Autodesk Fusion 360 part; units mm, degrees
(part 6 of 6)
equation "ChamberRear = CaseDepth - Cover - 2.8 mm" comment "Rear of closed sampling cartridge"
equation "ChamberLid = 2 mm" comment "Independent internal chamber lid"
equation "ChamberSideX = 45.6 mm" comment "Start of viewer-left vertical gas chamber column"
equation "ChamberLeft = 2.9 mm" comment "Upper chamber inner-case margin"
equation "ChamberRight = CaseWidth - 2.9 mm" comment "Upper and side chamber extent"
equation "ChamberBottom = 30 mm" comment "Lower gas column clears USB mounting region"
equation "ChamberTop = CaseHeight - 2.9 mm" comment "Top clearance to housing"
equation "ChamberBarY = 87 mm" comment "Lower edge of horizontal upper gas chamber"
equation "GasY = 105 mm" comment "Upper cross-flow port height"
equation "GasZ = 23 mm" comment "Side-fitting depth centre"
equation "GasBore = 2.5 mm" comment "5 mm ID nominal sample ports"
equation "UsbY = 16 mm" comment "Low on viewer-left side, below gas column"
equation "UsbZ = 27 mm" comment "USB connector centre depth"
equation "ButtonY = 45 mm" comment "Right-side power button, behind holder"
equation "ButtonZ = 44.5 mm" comment "Button clearance behind measured thin holder"
equation "d45 = CaseWidth"
equation "d46 = CaseHeight"
equation "d47 = CaseDepth - Cover"
equation "d49 = RearInset"
equation "d50 = RearInset"
equation "d51 = CaseWidth - 2 * RearInset"
equation "d52 = CaseHeight - 2 * RearInset"
equation "d54 = CornerRadius"
equation "d57 = Wall"
equation "d58 = Wall"
equation "d59 = CaseWidth - 2 * Wall"
equation "d60 = CaseHeight - 2 * Wall"
equation "d61 = CaseDepth"
equation "d64 = CornerRadius - Wall"
equation "d67 = DisplayX - DisplayFit"
equation "d68 = DisplayY - DisplayFit"
equation "d69 = DisplayWidth + 2 * DisplayFit"
equation "d70 = DisplayHeight + 2 * DisplayFit"
equation "d75 = -( -( GasZ ) )"
equation "d76 = GasY"
equation "d78 = CaseWidth + 2 mm"
equation "d82 = -( -( ButtonZ ) )"
equation "d83 = ButtonY"
equation "d85 = Wall + 2 mm"
equation "d87 = CaseWidth - Wall - 1 mm"
equation "d89 = -( -( ( UsbZ - 8 mm ) + ( 16 mm ) ) )"
equation "d90 = UsbY - 10 mm"
equation "d93 = Wall + 2 mm"
equation "d95 = CaseDepth - Cover + CoverGap"
equation "d97 = RearInset"
equation "d98 = RearInset"
equation "d99 = CaseWidth - 2 * RearInset"
equation "d100 = CaseHeight - 2 * RearInset"
equation "d101 = Cover - CoverGap"
equation "d104 = CornerRadius"
equation "d105 = DisplayFront"
equation "d107 = DisplayX"
equation "d108 = DisplayY"
equation "d109 = DisplayWidth"
equation "d110 = DisplayHeight"
equation "d111 = DisplayDepth"
equation "d115 = DisplayFront + 3 mm"
equation "d117 = CaseWidth / 2 - 32.7 mm"
equation "d118 = CaseHeight / 2 - 54 mm"
equation "d123 = DisplayFront - 0.1 mm"
equation "d125 = ( CaseWidth - GlassWidth ) / 2"
equation "d126 = ( CaseHeight - GlassHeight ) / 2"
equation "d127 = GlassWidth"
equation "d128 = GlassHeight"
equation "d131 = DisplayFront"
equation "d133 = ( CaseWidth - GlassWidth ) / 2"
equation "d134 = ( CaseHeight - GlassHeight ) / 2"
equation "d135 = GlassWidth"
equation "d136 = GlassHeight"
equation "d139 = DisplayFront - 0.1 mm"
equation "d141 = ( CaseWidth - ActiveWidth ) / 2"
equation "d142 = ( CaseHeight - ActiveHeight ) / 2"
equation "d143 = ActiveWidth"
equation "d144 = ActiveHeight"
equation "d147 = DisplayFront"
equation "d149 = ( CaseWidth - ActiveWidth ) / 2"
equation "d150 = ( CaseHeight - ActiveHeight ) / 2"
equation "d151 = ActiveWidth"
equation "d152 = ActiveHeight"
equation "d157 = CaseWidth / 2 - 32.53 mm"
equation "d158 = CaseHeight / 2 - 54 mm"
equation "d165 = CaseWidth / 2 - 30 mm"
equation "d166 = CaseHeight / 2 - 51.3 mm"
equation "d172 = CaseWidth / 2 - 30 mm"
equation "d173 = CaseHeight / 2 + 51.3 mm"
equation "d179 = CaseWidth / 2 + 30 mm"
equation "d180 = CaseHeight / 2 - 51.3 mm"
equation "d186 = CaseWidth / 2 + 30 mm"
equation "d187 = CaseHeight / 2 + 51.3 mm"
equation "d193 = 15 mm + DisplayX - 2.85 mm"
equation "d194 = 75 mm + DisplayY - 4.1 mm"
equation "d201 = 47 mm + DisplayX - 2.85 mm"
equation "d202 = 90 mm + DisplayY - 4.1 mm"
equation "d209 = 34 mm + DisplayX - 2.85 mm"
equation "d210 = 79 mm + DisplayY - 4.1 mm"
equation "d217 = 14 mm + DisplayX - 2.85 mm"
equation "d218 = 18 mm + DisplayY - 4.1 mm"
equation "d225 = 24 mm + DisplayX - 2.85 mm"
equation "d226 = 23 mm + DisplayY - 4.1 mm"
equation "d233 = 30 mm + DisplayX - 2.85 mm"
equation "d234 = 9 mm + DisplayY - 4.1 mm"
equation "d241 = 23 mm + DisplayX - 2.85 mm"
equation "d242 = 62 mm + DisplayY - 4.1 mm"
equation "d249 = 52 mm + DisplayX - 2.85 mm"
equation "d250 = 34 mm + DisplayY - 4.1 mm"
equation "d257 = CaseDepth - 13 mm"
equation "d264 = CaseDepth - 9.85 mm"
equation "d271 = CaseDepth - 3.65 mm"
equation "d278 = CaseDepth - 3.75 mm"
equation "d285 = CaseDepth - 1.65 mm"
equation "d292 = CaseDepth - 13 mm"
equation "d294 = CaseWidth - 6 mm"
equation "d299 = CaseDepth - 9.85 mm"
equation "d301 = CaseWidth - 6 mm"
equation "d306 = CaseDepth - 3.65 mm"
equation "d308 = CaseWidth - 6 mm"
equation "d313 = CaseDepth - 3.75 mm"
equation "d315 = CaseWidth - 6 mm"
equation "d320 = CaseDepth - 1.65 mm"
equation "d322 = CaseWidth - 6 mm"
equation "d327 = CaseDepth - 13 mm"
equation "d330 = CaseHeight - 6 mm"
equation "d334 = CaseDepth - 9.85 mm"
equation "d337 = CaseHeight - 6 mm"
equation "d341 = CaseDepth - 3.65 mm"
equation "d344 = CaseHeight - 6 mm"
equation "d348 = CaseDepth - 3.75 mm"
equation "d351 = CaseHeight - 6 mm"
equation "d355 = CaseDepth - 1.65 mm"
equation "d358 = CaseHeight - 6 mm"
equation "d362 = CaseDepth - 13 mm"
equation "d364 = CaseWidth - 6 mm"
equation "d365 = CaseHeight - 6 mm"
equation "d369 = CaseDepth - 9.85 mm"
equation "d371 = CaseWidth - 6 mm"
equation "d372 = CaseHeight - 6 mm"
equation "d376 = CaseDepth - 3.65 mm"
equation "d378 = CaseWidth - 6 mm"
equation "d379 = CaseHeight - 6 mm"
equation "d383 = CaseDepth - 3.75 mm"
equation "d385 = CaseWidth - 6 mm"
equation "d386 = CaseHeight - 6 mm"
equation "d390 = CaseDepth - 1.65 mm"
equation "d392 = CaseWidth - 6 mm"
equation "d393 = CaseHeight - 6 mm"
equation "d435 = HolderZ"
equation "d437 = HolderX"
equation "d438 = HolderY"
equation "d439 = HolderWidth"
equation "d440 = HolderHeight"
equation "d441 = HolderDepth"
equation "d445 = HolderZ + 1.1 mm"
equation "d447 = HolderX + 1 mm"
equation "d448 = HolderY + 2 mm"
equation "d449 = HolderWidth - 2 mm"
equation "d450 = HolderHeight - 4 mm"
equation "d451 = HolderDepth"
equation "d453 = HolderY + 5 mm"
equation "d455 = HolderX + 10.8 mm"
equation "d456 = -( -( HolderZ + 10.25 mm ) )"
equation "d460 = HolderY + 5 mm"
equation "d462 = HolderX + 31.2 mm"
equation "d463 = -( -( HolderZ + 10.25 mm ) )"
equation "d793 = -( -( ButtonZ ) )"
equation "d794 = ButtonY"
equation "d800 = -( -( ButtonZ ) )"
equation "d801 = ButtonY"
equation "d807 = -( -( ( ButtonZ - 4 mm ) + ( 8 mm ) ) )"
equation "d808 = ButtonY - 4 mm"
equation "d815 = -( -( ButtonZ ) )"
equation "d816 = ButtonY"
equation "d820 = CaseDepth - 3.75 mm"
equation "d827 = CaseDepth - 3.75 mm"
equation "d830 = CaseHeight - 6 mm"
equation "d834 = CaseDepth - 3.75 mm"
equation "d836 = CaseWidth - 6 mm"
equation "d841 = CaseDepth - 3.75 mm"
equation "d843 = CaseWidth - 6 mm"
equation "d844 = CaseHeight - 6 mm"
equation "d850 = CaseDepth"
equation "d858 = CaseDepth - 4.4 mm"
equation "d864 = CaseWidth - 6 mm"
equation "d866 = CaseDepth"
equation "d873 = CaseHeight - 6 mm"
equation "d874 = CaseDepth"
equation "d880 = CaseWidth - 6 mm"
equation "d881 = CaseHeight - 6 mm"
equation "d882 = CaseDepth"
equation "d888 = CaseWidth - 6 mm"
equation "d890 = CaseDepth - 4.4 mm"
equation "d897 = CaseHeight - 6 mm"
equation "d898 = CaseDepth - 4.4 mm"
equation "d904 = CaseWidth - 6 mm"
equation "d905 = CaseHeight - 6 mm"
equation "d906 = CaseDepth - 4.4 mm"
equation "d912 = CaseWidth - 2.4 mm"
equation "d914 = -( -( ( 19.25 mm ) + ( 15.5 mm ) ) )"
equation "d920 = CaseWidth - 4.4 mm"
equation "d922 = -( -( ( 17 mm ) + ( 20 mm ) ) )"
equation "d928 = CaseWidth - 4.5 mm"
equation "d930 = -( -( ( 23.5 mm ) + ( 7 mm ) ) )"
equation "d936 = CaseWidth - 2.5 mm"
equation "d938 = -( -( ( 23.5 mm ) + ( 7 mm ) ) )"
equation "d944 = CaseWidth - 1.91 mm"
equation "d948 = CaseWidth - 1.91 mm"
equation "d952 = CaseWidth - 1.73 mm"
equation "d956 = CaseWidth - 1.23 mm"
equation "d958 = CaseWidth - 0.1 mm"
equation "d962 = CaseWidth - 14.9 mm"
equation "d970 = CaseWidth - 11.3 mm"
equation "d977 = CaseWidth - 11.3 mm"
equation "d984 = CaseWidth - 17.5 mm"
equation "d992 = CaseWidth - 15.5 mm"
equation "d999 = CaseWidth - 15.5 mm"
equation "d1004 = CaseWidth - 6.4 mm"
equation "d1006 = -( -( 21.25 mm ) )"
equation "d1011 = CaseWidth - 6.5 mm"
equation "d1013 = -( -( 21.25 mm ) )"
equation "d1018 = CaseWidth - 2.5 mm"
equation "d1020 = -( -( 21.25 mm ) )"
equation "d1025 = CaseWidth - 6.4 mm"
equation "d1032 = CaseWidth - 6.5 mm"
equation "d1039 = CaseWidth - 2.5 mm"
equation "d1048 = CaseWidth - 18 mm"
equation "d1056 = CaseWidth - 8.7 mm"
equation "d1064 = CaseWidth - 11.3 mm"
equation "d1071 = CaseWidth - 15.5 mm"
equation "d1076 = CaseWidth - 7.5 mm"
equation "d1080 = CaseWidth - 2.1 mm"
equation "d1084 = CaseWidth - 7.6 mm"
equation "d1088 = CaseWidth - 2.2 mm"
equation "d1094 = CaseWidth - 7.2 mm"
equation "d1102 = CaseWidth - 7.2 mm"
equation "d1110 = CaseWidth - 5.2 mm"
equation "d1118 = CaseWidth - 5.2 mm"
equation "d1124 = CaseWidth - 7.6 mm"
equation "d1130 = CaseWidth - 6.6 mm"
equation "d1136 = CaseWidth - 1.70 mm"
equation "d1140 = CaseWidth - 1.71 mm"
equation "d1146 = CaseWidth - 4.0 mm"
equation "d1154 = CaseWidth - 4.0 mm"
equation "d1162 = CaseWidth - 4.0 mm"
equation "d1170 = CaseWidth - 4.0 mm"
equation "d1178 = CaseWidth - 4.0 mm"
equation "d1186 = CaseWidth - 4.0 mm"
equation "d1194 = CaseWidth - 4.0 mm"
equation "d1202 = CaseWidth - 4.0 mm"
equation "d1210 = CaseWidth - 4.0 mm"
equation "d1218 = CaseWidth - 4.0 mm"
equation "d1226 = CaseWidth - 4.0 mm"
equation "d1234 = CaseWidth - 4.0 mm"
equation "d1242 = CaseWidth - 4.0 mm"
equation "d1250 = CaseWidth - 4.0 mm"
equation "d1258 = CaseWidth - 4.0 mm"
equation "d1266 = CaseWidth - 4.0 mm"
equation "d1306 = CaseWidth - 5 mm"
equation "d1313 = CaseWidth - 5.7 mm"
equation "d1320 = CaseWidth - 9.3 mm"
equation "d1328 = CaseWidth - 6.6 mm"
equation "d1336 = CaseWidth - 5.7 mm"
equation "d1607 = ChamberRear - ChamberLid"
equation "d1609 = ChamberLeft"
equation "d1610 = ChamberBarY"
equation "d1611 = ( ChamberRight ) - ( ChamberLeft )"
equation "d1612 = ( ChamberTop ) - ( ChamberBarY )"
equation "d1613 = ChamberLid"
equation "d1615 = ChamberRear - ChamberLid"
equation "d1617 = ChamberSideX"
equation "d1618 = ChamberBottom"
equation "d1619 = ( ChamberRight ) - ( ChamberSideX )"
equation "d1620 = ( ChamberTop ) - ( ChamberBottom )"
equation "d1621 = ChamberLid"
equation "d1625 = ChamberFront - 1 mm"
equation "d1628 = CaseHeight - 6 mm"
equation "d1630 = 2 * CaseDepth"
equation "d1632 = ChamberFront - 1 mm"
equation "d1634 = CaseWidth - 6 mm"
equation "d1635 = CaseHeight - 6 mm"
equation "d1637 = 2 * CaseDepth"
equation "d1639 = ChamberFront - 1 mm"
equation "d1641 = ChamberLeft - 1 mm"
equation "d1643 = 18.1 mm - ( ChamberLeft - 1 mm )"
equation "d1644 = CaseHeight - 114.8 mm"
equation "d1645 = 2 * CaseDepth"
equation "d1647 = ChamberRear - ChamberLid - 0.1 mm"
equation "d1652 = ChamberLid + 0.2 mm"
equation "d1654 = ChamberRear - ChamberLid - 0.1 mm"
equation "d1659 = ChamberLid + 0.2 mm"
equation "d1661 = ChamberRear - ChamberLid - 0.1 mm"
equation "d1666 = ChamberLid + 0.2 mm"
equation "d1668 = ChamberRear - ChamberLid - 0.1 mm"
equation "d1673 = ChamberLid + 0.2 mm"
equation "d1675 = ChamberRear - ChamberLid - 0.1 mm"
equation "d1680 = ChamberLid + 0.2 mm"
equation "d1682 = ChamberRear - ChamberLid - 0.1 mm"
equation "d1687 = ChamberLid + 0.2 mm"
equation "d1689 = ChamberRear - ChamberLid - 0.1 mm"
equation "d1694 = ChamberLid + 0.2 mm"
equation "d1696 = ChamberRear - ChamberLid - 0.1 mm"
equation "d1701 = ChamberLid + 0.2 mm"
equation "d1724 = ChamberRear - ChamberLid - 2 mm - 14.3 mm"
equation "d1726 = ChamberRear - ChamberLid - 6 mm"
equation "d1738 = ChamberRear - ChamberLid - 2 mm - 14.3 mm"
equation "d1740 = ChamberRear - ChamberLid - 6 mm"
equation "d1749 = -( -( ChamberFront + 17.15 mm ) )"
equation "d1756 = -( -( ChamberFront + 17.15 mm ) )"
equation "d1761 = ChamberFront + 12.15 mm"
equation "d1769 = ChamberFront + 2.5 mm"
equation "d1777 = ChamberFront + 2.5 mm"
equation "d1785 = ChamberFront + 2.5 mm"
equation "d1793 = ChamberFront + 25.5 mm"
equation "d1801 = ChamberRight - ChamberWall"
equation "d1803 = -( -( GasZ ) )"
equation "d1804 = GasY"
equation "d1806 = CaseWidth + 6 mm - ( ChamberRight - ChamberWall )"
equation "d1808 = ( ChamberRight - ChamberWall ) - 0.1 mm"
equation "d1810 = -( -( GasZ ) )"
equation "d1811 = GasY"
equation "d1812 = GasBore"
equation "d1813 = ( CaseWidth + 6 mm - ( ChamberRight - ChamberWall ) ) + 0.2 mm"
equation "d1817 = -( -( GasZ ) )"
equation "d1818 = GasY"
equation "d1820 = ChamberLeft + ChamberWall + 6 mm"
equation "d1822 = ( -6 mm ) - 0.1 mm"
equation "d1824 = -( -( GasZ ) )"
equation "d1825 = GasY"
equation "d1826 = GasBore"
equation "d1827 = ( ChamberLeft + ChamberWall + 6 mm ) + 0.2 mm"
equation "d1831 = -( -( 44.5 mm ) )"
equation "d1838 = -( -( 44.5 mm ) )"
equation "d1843 = ChamberFront + 2.5 mm"
equation "d1853 = -( -( ChamberFront + 15.2 mm ) )"
equation "d1858 = ChamberFront + 11 mm"
equation "d1866 = ChamberFront + 25.5 mm"
equation "d1874 = ChamberFront + 25.4 mm"
equation "d1881 = ChamberFront + 27.1 mm"
equation "d1888 = ChamberFront + 27.05 mm"
equation "d1895 = ChamberFront + 25.4 mm"
equation "d1902 = ChamberFront + 27.1 mm"
equation "d1909 = ChamberFront + 27.05 mm"
equation "d1916 = ChamberFront + 25.4 mm"
equation "d1923 = ChamberFront + 27.1 mm"
equation "d1930 = ChamberFront + 27.05 mm"
equation "d1937 = ChamberFront + 25.4 mm"
equation "d1944 = ChamberFront + 27.1 mm"
equation "d1951 = ChamberFront + 27.05 mm"
equation "d1958 = ChamberFront + 27.1 mm"
equation "d1966 = ChamberFront + 27.1 mm"
equation "d1974 = ChamberFront + 27.1 mm"
equation "d1982 = ChamberFront + 27.1 mm"
equation "d1992 = ChamberRear"
equation "d2000 = ChamberRear"
equation "d2008 = ChamberRear"
equation "d2016 = ChamberRear"
equation "d2024 = ChamberRear"
equation "d2032 = ChamberRear"
equation "d2040 = ChamberRear - ChamberLid"
equation "d2048 = ChamberRear - ChamberLid"
equation "d2056 = ChamberRear - ChamberLid"
equation "d2064 = ChamberRear - ChamberLid"
equation "d2072 = ChamberRear - ChamberLid"
equation "d2080 = ChamberRear - ChamberLid"
equation "d2088 = ChamberRear - ChamberLid"
equation "d2096 = ChamberRear - ChamberLid"
equation "d2104 = ChamberRear - ChamberLid - 2 mm"
equation "d2112 = ChamberRear - ChamberLid - 2 mm"
equation "d2120 = CaseWidth - 5.2 mm"
equation "d2128 = CaseWidth - 5.3 mm"
equation "d2136 = CaseWidth - 6 mm"
equation "d2143 = CaseWidth - 9.3 mm"
equation "d2151 = CaseWidth - 6.6 mm"
equation "d2159 = CaseWidth - 9.4 mm"
equation "d2165 = CaseWidth - 11.3 mm"
equation "d2175 = CaseWidth - 0.1 mm"
equation "d2186 = CaseWidth - 15.5 mm"
equation "d2194 = CaseWidth - 11.3 mm"
equation "d2202 = CaseWidth - 15.5 mm"
equation "d2212 = CaseWidth - 0.1 mm"
equation "d2225 = CaseWidth - 2.4 mm"
equation "d2238 = CaseWidth - 2.4 mm"
equation "d2257 = CaseWidth - 5.7 mm"
equation "d2265 = ChamberFront"
equation "d2267 = ChamberLeft"
equation "d2268 = ChamberBarY"
equation "d2269 = ( ChamberRight ) - ( ChamberLeft )"
equation "d2270 = ( ChamberTop ) - ( ChamberBarY )"
equation "d2271 = ChamberRear - ChamberLid - ChamberFront"
equation "d2273 = ChamberFront"
equation "d2275 = ChamberSideX"
equation "d2276 = ChamberBottom"
equation "d2277 = ( ChamberRight ) - ( ChamberSideX )"
equation "d2278 = ( ChamberTop ) - ( ChamberBottom )"
equation "d2279 = ChamberRear - ChamberLid - ChamberFront"
equation "d2281 = ChamberFront + ChamberWall"
equation "d2283 = ChamberLeft + ChamberWall"
equation "d2284 = ChamberBarY + ChamberWall"
equation "d2285 = ChamberRight - ChamberLeft - 2 * ChamberWall"
equation "d2286 = ChamberTop - ChamberBarY - 2 * ChamberWall"
equation "d2287 = CaseDepth"
equation "d2289 = ChamberFront + ChamberWall"
equation "d2291 = ChamberSideX + ChamberWall"
equation "d2292 = ChamberBottom + ChamberWall"
equation "d2293 = ChamberRight - ChamberSideX - 2 * ChamberWall"
equation "d2294 = ChamberTop - ChamberBottom - 2 * ChamberWall"
equation "d2295 = CaseDepth"
equation "d2297 = ChamberFront"
equation "d2300 = CaseHeight - 6 mm"
equation "d2302 = ChamberRear - ChamberLid - ChamberFront"
equation "d2304 = ChamberFront"
equation "d2306 = CaseWidth - 6 mm"
equation "d2307 = CaseHeight - 6 mm"
equation "d2309 = ChamberRear - ChamberLid - ChamberFront"
equation "d2311 = ChamberFront"
equation "d2313 = ChamberLeft"
equation "d2315 = 20.1 mm - ChamberLeft"
equation "d2316 = ChamberTop - 112.8 mm"
equation "d2317 = ChamberRear - ChamberLid - ChamberFront"
equation "d2319 = ChamberFront"
equation "d2324 = ChamberRear - ChamberLid - ChamberFront"
equation "d2326 = ChamberFront"
equation "d2331 = ChamberRear - ChamberLid - ChamberFront"
equation "d2333 = ChamberFront - 1 mm"
equation "d2335 = -( ChamberLeft - 10 mm )"
equation "d2336 = -( -10 mm )"
equation "d2338 = CaseHeight + 20 mm"
equation "d2339 = 2 * CaseDepth"
equation "d2341 = ChamberFront - 1 mm"
equation "d2343 = ChamberRight"
equation "d2344 = -( -10 mm )"
equation "d2346 = CaseHeight + 20 mm"
equation "d2347 = 2 * CaseDepth"
equation "d2349 = ChamberFront - 1 mm"
equation "d2351 = -( ChamberLeft - 10 mm )"
equation "d2352 = ChamberTop"
equation "d2353 = ChamberRight - ChamberLeft + 20 mm"
equation "d2355 = 2 * CaseDepth"
equation "d2359 = ChamberFront - 1 mm"
equation "d2362 = CaseHeight - 6 mm"
equation "d2364 = 2 * CaseDepth"
equation "d2366 = ChamberFront - 1 mm"
equation "d2368 = CaseWidth - 6 mm"
equation "d2369 = CaseHeight - 6 mm"
equation "d2371 = 2 * CaseDepth"
equation "d2373 = ChamberFront - 1 mm"
equation "d2375 = ChamberLeft - 1 mm"
equation "d2377 = 18.1 mm - ( ChamberLeft - 1 mm )"
equation "d2378 = CaseHeight - 114.8 mm"
equation "d2379 = 2 * CaseDepth"
equation "d2381 = ChamberFront - 0.1 mm"
equation "d2386 = ChamberRear - ChamberLid - 2 mm - ( ChamberFront - 0.1 mm )"
equation "d2388 = ChamberRear - ChamberLid - 2.1 mm"
equation "d2395 = ChamberFront - 0.1 mm"
equation "d2400 = ChamberRear - ChamberLid - 2 mm - ( ChamberFront - 0.1 mm )"
equation "d2402 = ChamberRear - ChamberLid - 2.1 mm"
equation "d2409 = ChamberRear - ChamberLid - 6 mm"
equation "d2417 = ChamberRear - ChamberLid - 6 mm"
equation "d2424 = ChamberRear - ChamberLid - 4 mm"
equation "d2431 = ChamberRear - ChamberLid - 6 mm"
equation "d2439 = ChamberRear - ChamberLid - 6 mm"
equation "d2446 = ChamberRear - ChamberLid - 4 mm"
equation "d2453 = ChamberRear - ChamberLid - 6 mm"
equation "d2461 = ChamberRear - ChamberLid - 6 mm"
equation "d2468 = ChamberRear - ChamberLid - 4 mm"
equation "d2475 = ChamberRear - ChamberLid - 6 mm"
equation "d2483 = ChamberRear - ChamberLid - 6 mm"
equation "d2490 = ChamberRear - ChamberLid - 4 mm"
equation "d2497 = ChamberRear - ChamberLid - 6 mm"
equation "d2505 = ChamberRear - ChamberLid - 6 mm"
equation "d2512 = ChamberRear - ChamberLid - 4 mm"
equation "d2519 = ChamberRear - ChamberLid - 6 mm"
equation "d2527 = ChamberRear - ChamberLid - 6 mm"
equation "d2534 = ChamberRear - ChamberLid - 4 mm"
equation "d2543 = -( -( GasZ ) )"
equation "d2544 = GasY"
equation "d2546 = CaseWidth + 2 mm"
equation "d2550 = -( -( 44.5 mm ) )"
equation "d2555 = CaseWidth - 5.7 mm"
named bodies: "Tapered housing", "Single screw-fastened rear cover", "Guition retained factory frame", "Black border glass", "480x800 active area", "Guition PCB outline reference", "ESP32-P4 visual reference", "ESP32-C6 radio module reference", "Memory package reference", "Power inductor reference", "Board IC reference", "Rear USB connector reference", "Display FPC latch reference", "Expansion header reference", "GEN-M3-BHCS-L8-AF2 — joined head and shaft", "GEN-M3-HEATSET-OD4.2-L5 — hollow simplified insert", "Measured occupied holder outer frame", "18650 reference cylinder - 18.2 diameter x 69 length", "Red battery disconnect reference body", "Red battery disconnect mating reference", "Shaped electronics carrier", "Reshaped future PCB", "Power-stage allocation", "Analog allocation", "Digital allocation", "GEN-M2-SHCS-L7-AF1.5 — joined head and shaft", "GEN-M2-HEATSET-OD3.2-L4 — hollow simplified insert", "lower clip screw seat", "upper clip screw seat", "GEN-M2-SHCS-L5-AF1.5 — joined head and shaft", "12 mm button barrel", "External button bezel", "Button terminal block allowance", "Green 1NO button face", "Metal panel insert with 0.25 mm perimeter clearance", "Interior printed USB backing flange", "USB 0.60 mm daughterboard", "USB stainless shell body reference", "Insulator rear block — visual reference", "LIM gasket nominal reference", "USB contact visual stripe", "USB contact visual stripe (1)", "USB contact visual stripe (2)", "USB contact visual stripe (3)", "USB contact visual stripe (4)", "USB contact visual stripe (5)", "USB contact visual stripe (6)", "USB contact visual stripe (7)", "USB contact visual stripe (8)", "USB contact visual stripe (9)", "USB contact visual stripe (10)", "USB contact visual stripe (11)", "USB contact visual stripe (12)", "USB contact visual stripe (13)", "USB contact visual stripe (14)", "USB contact visual stripe (15)", "GEN-M2-SHCS-L4-AF1.5 — joined head and shaft", "GEN-M2-SHCS-L6-AF1.5 — joined head and shaft", "USB rear clamp strap", "Internal L lid", "AO2 full-size body", "AO2 connector allowance", "ZE07-CO rotated total envelope", "MD62 rotated body envelope", "MD62 27 mm lead allowance", "GYBMEP wired module envelope", "left inlet hollow fitting", "right exhaust hollow fitting", "Harness feedthrough envelope", "ZE07-CO PCB — drawing-derived stack", "ZE07-CO sensor can — Ø20 x 16.7 reference", "ZE07 opposite-side pin header allowance — profile unmeasured", "GYBMEP board — provisional visual reference", "Illustrative I2C plated pad", "Illustrative I2C plated pad (1)", "Illustrative I2C plated pad (2)", "Illustrative I2C plated pad (3)", "Humidity metal cap — placement unverified", "Regulator allocation visual", "Interface IC visual", "Passive component reference", "USB outside-cavity corner trim tool", "Closed-wall L cartridge — unqualified sealing concept"
